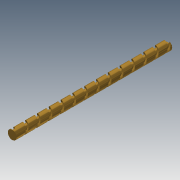
# Autodesk Inventor part: Part1
Saved by Autodesk Inventor 2014 SP1 (Build 180222100, 222)
## iProperties
Created: 2014-03-24
Part Number: Part1
Material: Generic
Document SubType Name: Modeling
Designer: tom
Density: 1 g/cm^3
Appearance: Brass - Satin
Author: tom
Autodesk Inventor part; units mm, degrees
ref_plane "YZ Plane" through (0, 0, 0) normal (1, 0, 0) x (0, 1, 0)
ref_plane "XZ Plane" through (0, 0, 0) normal (0, 1, 0) x (-1, 0, 0)
ref_plane "XY Plane" through (0, 0, 0) normal (0, 0, 1) x (1, 0, 0)
sketch "Sketch1" plane through (0, 0, 0) normal (0, 0, 1) x (1, 0, 0)
  circle A0 centre (0, 0) radius 1.5
  dimension "d0" = 3
  constraints: 1 centre point, 1 coincident
  measures "d0" diameter of A0
extrude "Extrusion1" add sketch "Sketch1" along normal blind 52.7
sketch "Sketch3" plane through (0, 0, 0) normal (1, 0, 0) x (0, 1, 0)
  line L0 (0.9, 0) -> (0.9, 1)
  line L1 (1.5, 1) -> (1.5, 0)
  line L2 (1.5, 0) -> (0.9, 0)
  line L3 (0.9, 0) -> (0.9, 1)
  line L4 (0.9, 1) -> (1.5, 1)
  line L5 (1.5, 0) -> (0.9, 0)
  line L6 (0, 0) -> (0, 1)
  line L7 (0.9, 52.7) -> (0.9, 51.7)
  line L8 (0.9, 51.7) -> (1.5, 51.7)
  line L9 (1.5, 51.7) -> (1.5, 52.7)
  line L10 (1.5, 52.7) -> (0.9, 52.7)
  line L11 (1.5, 51.7) -> (0.9, 51.7)
  dimension "d7" = 0.9
  dimension "d8" = 1
  dimension "d9" = 1
  constraints: 24 end point, 4 equal length, 3 perpendicular
  measures "d7" distance of L6.start L0.start
  measures "d8" distance of L0.start L0.end
  measures "d9" distance of L7.start L7.end
coil "Coil1" sketch "Sketch3" operation cut axis through (0, 0, 0) along (0, 0, -1) pitch 4 turns 30 hand left contours L10 L9 L8 L7
body "Solid1"
